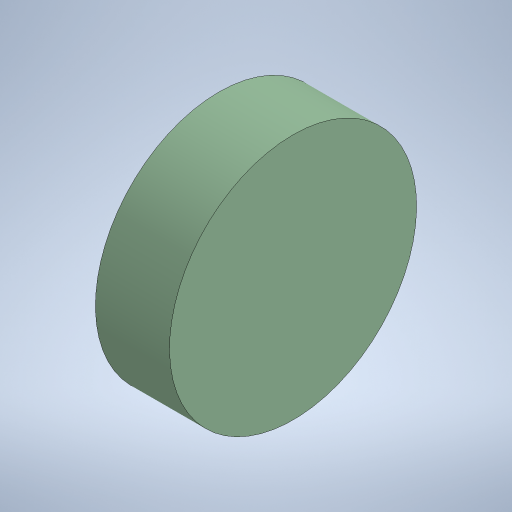
# Autodesk Inventor part: Temp - Wheel
Saved by Autodesk Inventor 2023.2 (Build 272271000, 271)
## iProperties
Created: 2023-11-13
Part Number: Temp - Wheel
Material: Silicon Nitride
Document SubType Name: Modeling
Designer: Nathan Cai
Density: 3.18 g/cm^3
Appearance: Rubber - Green
Mass: 23.9811 g
Surface Area: 25.3354 cm^2
Volume: 7.54123 cm^3
Author: Nathan Cai
Autodesk Inventor part; units mm, degrees
ref_plane "YZ Plane" through (0, 0, 0) normal (1, 0, 0) x (0, 1, 0)
ref_plane "XZ Plane" through (0, 0, 0) normal (0, 1, 0) x (-1, 0, 0)
ref_plane "XY Plane" through (0, 0, 0) normal (0, 0, 1) x (1, 0, 0)
sketch "Sketch1" plane through (0, 0, 0) normal (1, 0, 0) x (0, 1, 0)
  circle A0 centre (0, 0) radius 15.875
  circle A1 centre (0, 0) radius 3.175
  dimension "d0" = 31.75
  dimension "d5" = 6.35
  constraints: 2 centre point, 2 coincident
  measures "d0" diameter of A0
  measures "d5" diameter of A1
extrude "Extrusion1" add sketch "Sketch1" along normal blind 9.525 contours A0 | A1
body "Solid1"
